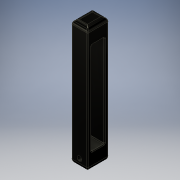
# Autodesk Inventor part: PhoneBracketBottom
Saved by Autodesk Inventor 2018 (Build 220112000, 112)
## iProperties
Created: 2018-08-29
Part Number: PhoneBracketBottom
Material: Generic
Document SubType Name: Modeling
Designer: anirudh
Density: 1 g/cm^3
Appearance: Gunmetal
Author: anirudh
Autodesk Inventor part; units mm, degrees
ref_plane "Work Plane1" through (0, 0, 0) normal (0, 0, -1) x (-1, 0, 0)
sketch "Sketch2" plane through (0, 0, 0) normal (0, 0, -1) x (-1, 0, 0)
  line L0 (-145.415, 72.39) -> (0, 72.39) projected
  line L1 (-145.415, 72.39) -> (-132.715, 72.39)
  line L2 (-132.715, 72.39) -> (-132.715, 85.09)
  line L3 (-132.715, 85.09) -> (-120.015, 85.09)
  line L4 (-120.015, 85.09) -> (-120.015, 72.39)
  line L5 (-120.015, 72.39) -> (-132.715, 72.39)
  line L6 (0, 0) -> (-145.415, 0) projected
  line L7 (-145.415, 0) -> (-132.715, 0)
  line L8 (-132.715, 0) -> (-120.015, 0)
  line L9 (-120.015, 0) -> (-120.015, -12.7)
  line L10 (-120.015, -12.7) -> (-132.715, -12.7)
  line L11 (-132.715, -12.7) -> (-132.715, 0)
  dimension "d4" = 12.7
  dimension "d5" = 12.7
  dimension "d6" = 12.7
  dimension "d7" = 12.7
  dimension "d8" = 12.7
  dimension "d9" = 12.7
  constraints: 20 end point, 4 perpendicular, 3 equal length, 3 point on line, 1 horizontal
  measures "d4" distance of L0.start L1.end
  measures "d5" distance of L1.end L2.end
  measures "d6" distance of L2.end L3.end
  measures "d7" distance of L6.end L7.end
  measures "d8" distance of L9.end L10.end
  measures "d9" distance of L8.end L9.end
extrude "Extrusion2" add sketch "Sketch2" against normal blind 10.16
ref_plane "Work Plane3" through (0, 0, 10.16) normal (0, 0, 1) x (1, 0, 0)
sketch "Sketch3" plane through (0, 0, 10.16) normal (0, 0, 1) x (1, 0, 0)
  line L0 (132.715, 85.09) -> (120.015, 85.09) projected
  line L1 (132.715, -12.7) -> (132.715, 0) projected
  line L2 (120.015, 85.09) -> (132.715, 85.09)
  line L3 (132.715, 85.09) -> (132.715, -12.7)
  line L4 (132.715, -12.7) -> (120.015, -12.7)
  line L5 (120.015, -12.7) -> (120.015, 85.09)
  point P0 (0, 0)
  constraints: 8 end point, 2 parallel, 1 horizontal, 1 perpendicular
extrude "Extrusion3" add sketch "Sketch3" along normal blind 3.175
ref_plane "Work Plane2" through (0, 0, 0) normal (0, 0, -1) x (-1, 0, 0)
sketch "Sketch4" plane through (0, 0, 0) normal (0, 0, -1) x (-1, 0, 0)
  line L0 (-120.015, 85.09) -> (-132.715, 85.09) projected
  line L1 (-120.015, -12.7) -> (-120.015, 0) projected
  line L2 (-132.715, 85.09) -> (-120.015, 85.09)
  line L3 (-120.015, 85.09) -> (-120.015, -12.7)
  line L4 (-120.015, -12.7) -> (-132.715, -12.7)
  line L5 (-132.715, -12.7) -> (-132.715, 85.09)
  point P0 (0, 0)
  constraints: 8 end point, 2 parallel, 1 horizontal, 1 perpendicular
extrude "Extrusion4" add sketch "Sketch4" along normal blind 3.175
ref_plane "Work Plane4" through (0, 0, 13.335) normal (0, 0, 1) x (1, 0, 0)
sketch "Sketch5" plane through (0, 0, 13.335) normal (0, 0, 1) x (1, 0, 0)
  line L0 (132.715, -12.7) -> (119.9435, -12.7)
  circle A0 centre (126.3292, -6.35) radius 1.85
  point P0 (0, 0)
  dimension "d16" = 3.7
  constraints: 2 end point, 1 centre point
  measures "d16" diameter of A0
extrude "Extrusion5" cut sketch "Sketch5" against normal blind 68.2625
fillet "Fillet1" radius 3.175 8 edges at (126.365, 85.09, 13.335) (120.015, 85.09, 5.08) (126.365, 85.09, -3.175) (132.715, 85.09, 5.08) (126.365, -12.7, 13.335) (132.715, -12.7, 5.08) (126.365, -12.7, -3.175) (120.015, -12.7, 5.08)
fillet "Fillet2" radius 0.635 24 edges at (120.9449, 84.1601, -2.2451) (120.9449, -11.7701, -2.2451) (120.015, 36.195, -3.175) (120.015, 36.195, 0) (120.015, 72.39, 5.08) (120.015, 36.195, 10.16) (120.015, 0, 5.08) (120.9449, -11.7701, 12.4051) (120.9449, 84.1601, 12.4051) (120.015, 36.195, 13.335) (131.7851, 84.1601, 12.4051) (131.7851, -11.7701, 12.4051) (132.715, 36.195, 13.335) (131.7851, -11.7701, -2.2451) (131.7851, 84.1601, -2.2451) (132.715, 36.195, -3.175) (132.715, 72.39, 5.08) (132.715, 36.195, 10.16) (132.715, 36.195, 0) (132.715, 0, 5.08) (126.365, 0, 0) (126.365, 0, 10.16) (126.365, 72.39, 0) (126.365, 72.39, 10.16)
body "Solid1"
